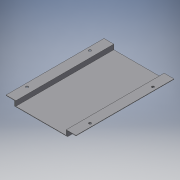
# Autodesk Inventor part: PCB-Mount
Saved by Autodesk Inventor 2016 SP2 (Build 200236200, 236)
## iProperties
Created: 2018-08-07
Part Number: PCB-Mount
Material: Generisch
Document SubType Name: Modeling
Designer: Nils
Density: 1 g/cm^3
Appearance: Vorgabe
Author: Nils
Autodesk Inventor part; units mm, degrees
ref_plane "YZ Plane" through (0, 0, 0) normal (1, 0, 0) x (0, 1, 0)
ref_plane "XZ Plane" through (0, 0, 0) normal (0, 1, 0) x (-1, 0, 0)
ref_plane "XY Plane" through (0, 0, 0) normal (0, 0, 1) x (1, 0, 0)
sketch "Skizze1" plane through (0, 0, 0) normal (0, 0, 1) x (1, 0, 0)
  line L0 (-90, 0) -> (-90, 36.75) construction
  line L1 (10, 0) -> (10, 36.75) construction
  line L2 (-90, 116.75) -> (-90, 147.085) construction
  line L3 (10, 147.085) -> (10, 116.75) construction
  circle A0 centre (-85, 121.75) radius 1.75 projected
  circle A1 centre (5, 121.75) radius 1.75 projected
  circle A2 centre (-85, 31.75) radius 1.75 projected
  circle A3 centre (5, 31.75) radius 1.75 projected
  line L4 (-90, 6.75) -> (10, 6.75)
  line L5 (10, 6.75) -> (10, 146.75)
  line L6 (10, 146.75) -> (-90, 146.75)
  line L7 (-90, 146.75) -> (-90, 6.75)
  point P0 (0, 0)
  dimension "d0" = 25
  dimension "d1" = 25
  constraints: 8 end point, 2 parallel, 2 point on line, 1 horizontal, 1 perpendicular
  measures "d0" distance from line of L6 A0.centre
  measures "d1" distance from line of L4 A2.centre
extrude "Extrusion1" add sketch "Skizze1" along normal blind 0.6
sketch "Skizze2" plane through (0, 0, 0) normal (0, 0, -1) x (-1, 0, 0)
  line L0 (90, 6.75) -> (-10, 6.75) projected
  line L1 (-10, 146.75) -> (90, 146.75) projected
  line L2 (2, 6.75) -> (78, 6.75)
  line L3 (78, 6.75) -> (78, 146.75)
  line L4 (78, 146.75) -> (2, 146.75)
  line L5 (2, 146.75) -> (2, 6.75)
  line L6 (-10, 6.75) -> (-10, 146.75) projected
  line L7 (90, 146.75) -> (90, 6.75) projected
  line L8 (78, 146.75) -> (2, 146.75)
  line L9 (2, 146.75) -> (2, 6.75)
  line L10 (2, 6.75) -> (78, 6.75)
  line L11 (78, 6.75) -> (78, 146.75)
  point P0 (0, 0)
  dimension "d4" = 12
  dimension "d5" = 12
  constraints: 16 end point, 4 parallel, 2 horizontal, 2 perpendicular, 2 point on line
  measures "d4" distance between parallel lines of L6 L5
  measures "d5" distance between parallel lines of L7 L3
extrude "Extrusion3" add sketch "Skizze2" along normal blind 7 contours L0 L5 L1 L3
sketch "Skizze3" plane through (0, 0, 0.6) normal (0, 0, 1) x (1, 0, 0)
  line L0 (-2, 6.75) -> (-78, 6.75) construction
  line L1 (-78, 6.75) -> (-78, 146.75) construction
  line L2 (-78, 146.75) -> (-2, 146.75) construction
  line L3 (-2, 146.75) -> (-2, 6.75) construction
  line L4 (-90, 6.75) -> (10, 6.75) projected
  line L5 (-78, 146.75) -> (-2, 146.75) projected
  line L6 (-4, 6.75) -> (-76, 6.75)
  line L7 (-76, 6.75) -> (-76, 146.75)
  line L8 (-76, 146.75) -> (-4, 146.75)
  line L9 (-4, 146.75) -> (-4, 6.75)
  point P0 (0, 0)
  dimension "d10" = 2
  dimension "d11" = 2
  constraints: 8 end point, 2 parallel, 2 point on line, 1 horizontal, 1 perpendicular
  measures "d10" distance between parallel lines of L1 L7
  measures "d11" distance between parallel lines of L3 L9
extrude "Extrusion4" cut sketch "Skizze3" against normal blind 7
